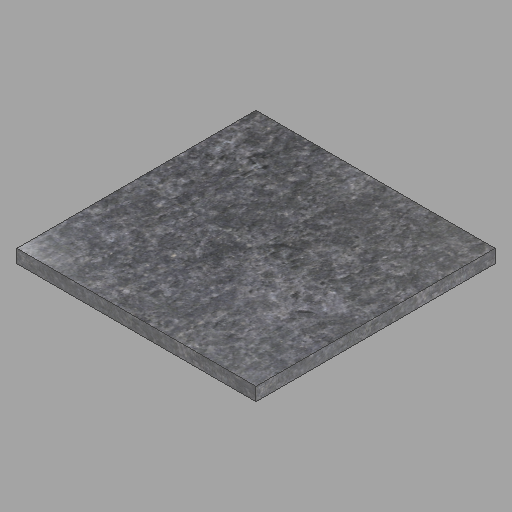
# Autodesk Inventor part: 18x18x2-77
Saved by Autodesk Inventor 2023 (Build 270158000, 158)
## iProperties
Created: 2022-03-01
Part Number: 18x18x2-77
Material: Granite, Cut, Polished
Document SubType Name: Modeling
Designer: awelt
Mass: 14335.4 g
Surface Area: 4645.15 cm^2
Volume: 5309.41 cm^3
Density: 2.7 g/cm^3
Appearance: Kasota SN sapphire
TEST: 0.0
Author: awelt
Autodesk Inventor part; units mm, degrees
ref_plane "YZ Plane" through (0, 0, 0) normal (1, 0, 0) x (0, 1, 0)
ref_plane "XZ Plane" through (0, 0, 0) normal (0, 1, 0) x (-1, 0, 0)
ref_plane "XY Plane" through (0, 0, 0) normal (0, 0, 1) x (1, 0, 0)
sketch "Sketch1" plane through (0, 0, 0) normal (0, 1, 0) x (-1, 0, 0)
  line L0 (228.6, -228.6) -> (-228.6, -228.6)
  line L1 (-228.6, -228.6) -> (-228.6, 228.6)
  line L2 (-228.6, 228.6) -> (228.6, 228.6)
  line L3 (228.6, 228.6) -> (228.6, -228.6)
  line L4 (228.6, -228.6) -> (-228.6, 228.6) construction
  line L5 (-228.6, -228.6) -> (228.6, 228.6) construction
  point P0 (0, 0)
  dimension "d0" = 457.2
  dimension "d1" = 457.2
  constraints: 12 end point, 2 midpoint, 2 parallel, 1 horizontal, 1 perpendicular
  measures "d0" distance of L1.end L2.end
  measures "d1" distance of L0.end L1.end
extrude "Extrusion1" add sketch "Sketch1" along normal blind 25.4
body "Solid1"
